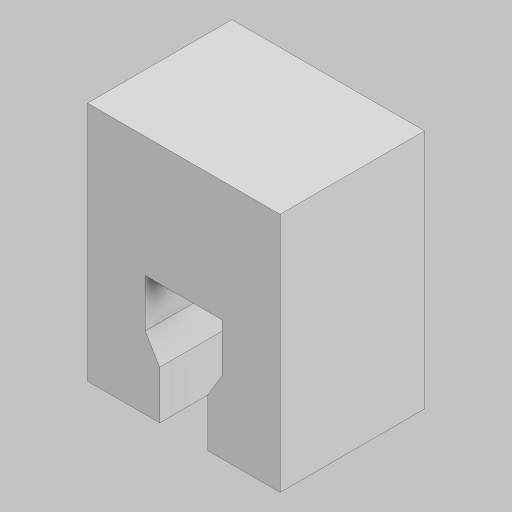
# Autodesk Inventor part: Bases_parametrizado
Saved by Autodesk Inventor 2023 (Build 270158000, 158)
## iProperties
Created: 2026-02-22
Part Number: Bases_parametrizado
Material: Genérico
Document SubType Name: Modeling
Designer: MARTIN MAESTRE
Density: 1 g/cm^3
Appearance: Valor por defecto
Author: MARTIN MAESTRE
Autodesk Inventor part; units mm, degrees
ref_plane "YZ Plane" through (0, 0, 0) normal (1, 0, 0) x (0, 1, 0)
ref_plane "XZ Plane" through (0, 0, 0) normal (0, 1, 0) x (-1, 0, 0)
ref_plane "XY Plane" through (0, 0, 0) normal (0, 0, 1) x (1, 0, 0)
sketch "Boceto1" plane through (0, 0, 0) normal (0, 0, 1) x (1, 0, 0)
  line L0 (0, 0) -> (40, 0)
  line L1 (40, 0) -> (40, 50)
  line L2 (40, 50) -> (0, 50)
  line L3 (0, 50) -> (0, 0)
  dimension "d0" = 40
  dimension "d1" = 50
  constraints: 8 end point, 2 parallel, 1 horizontal, 1 perpendicular
  measures "d0" distance of L2.end L1.end
  measures "d1" distance of L1.end L0.end
extrude "Extrusión1" add sketch "Boceto1" along normal blind 30
sketch "Boceto2" plane through (0, 0, 30) normal (0, 0, 1) x (1, 0, 0)
  line L0 (0, 0) -> (40, 0) projected
  line L1 (0, 0) -> (15, 0)
  line L2 (15, 0) -> (15, 10)
  line L3 (0, 0) -> (0, 25) construction
  line L4 (0, 50) -> (0, 0) construction
  line L5 (0, 25) -> (12, 25) construction
  line L6 (12, 25) -> (12, 15)
  line L7 (12, 15) -> (15, 10)
  line L8 (12, 25) -> (28, 25)
  line L9 (28, 25) -> (40, 25) construction
  line L10 (28, 25) -> (28, 15)
  line L11 (15, 0) -> (25, 0)
  line L12 (25, 0) -> (25, 10)
  line L13 (25, 10) -> (28, 15)
  dimension "d4" = 15
  dimension "d5" = 10
  dimension "d6" = 25
  dimension "d7" = 12
  dimension "d8" = 10
  dimension "d9" = 16
  dimension "d10" = 10
  dimension "d11" = 10
  dimension "d12" = 10
  constraints: 24 end point, 3 horizontal, 2 perpendicular, 2 point on line, 2 vertical, 1 midpoint
  measures "d4" distance of L0.start L1.end
  measures "d5" distance of L1.end L2.end
  measures "d6" distance of L0.start L3.end
  measures "d7" distance of L3.end L5.end
  measures "d8" distance of L5.end L6.end
  measures "d9" distance of L5.end L8.end
  measures "d10" distance of L8.end L10.end
  measures "d11" distance of L1.end L11.end
  measures "d12" distance of L11.end L12.end
extrude "Extrusión2" cut sketch "Boceto2" against normal blind 15
equation "\"Referencia_centro\" = 25"
